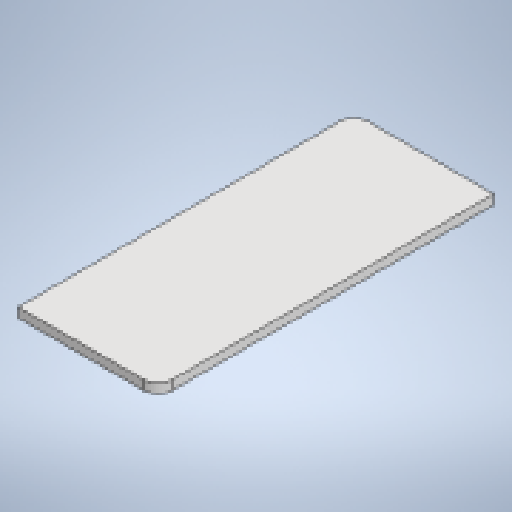
# Autodesk Inventor part: DS-B-104 ridge end cap
Saved by Autodesk Inventor 2025 (Build 290162010, 162A)
## iProperties
Created: 2025-01-16
Part Number: DS-B-104 ridge end cap
Material: Stainless Steel
Document SubType Name: Sheet Metal
Designer: pokla
Density: 8 g/cm^3
Sheet Metal Rule: AISI304 3mm Die 32
Appearance: Default
Mass: 77.6051 g
Surface Area: 103.045 cm^2
Volume: 9.70063 cm^3
Flat Pattern Width: 4.5 cm
Flat Pattern Length: 10.8 cm
Flat Pattern Area: 48.6 cm^2
Sheet Metal Width: 45,000 mm
Sheet Metal Length: 108,000 mm
Sheet Metal Area: 4860,000 mm^2
Author: pokla
Autodesk Inventor part; units mm, degrees
ref_plane "YZ Plane" through (0, 0, 0) normal (1, 0, 0) x (0, 1, 0)
ref_plane "XZ Plane" through (0, 0, 0) normal (0, 1, 0) x (-1, 0, 0)
ref_plane "XY Plane" through (0, 0, 0) normal (0, 0, 1) x (1, 0, 0)
sketch "Sketch1" plane through (0, 0, 0) normal (0, 0, 1) x (1, 0, 0)
  line L0 (-22.5, 54) -> (22.5, 54)
  line L1 (22.5, 54) -> (22.5, -54)
  line L2 (22.5, -54) -> (-22.5, -54)
  line L3 (-22.5, -54) -> (-22.5, 54)
  line L4 (-22.5, 54) -> (22.5, -54) construction
  point P0 (0, 0)
  point P1 (0, 0)
  dimension "d0" = 45
  dimension "d1" = 108
  measures "d0" distance of L0.start L0.end
  measures "d1" distance of L2.end L0.start
extrude "Plate1" add sketch "Sketch1" along normal blind 3
fillet "Corner Round2" radius 4.75 2 edges at (22.5, -54, 1.5) (-22.5, 54, 1.5)
equation "\"d0\" = RIDGE_1_width"
equation "\"d2\" = Thickness"
equation "\"BendReliefWidth\" = Thickness"
equation "\"BendReliefDepth\" = 0.5 * Thickness"
equation "\"CornerReliefSize\" = 4 * Thickness"
equation "\"MinimumRemnant\" = 2 * Thickness"
equation "\"TransitionRadius\" = BendRadius"
equation "\"JacobiRadiusSize\" = BendRadius"
equation "\"GapSize\" = Thickness"
equation "\"RIDGE_1_width\" = 45"
equation "\"Thickness\" = 3"
equation "\"BendRadius\" = 5"
body "Solid1"
